Autodesk Inventor part; units mm, degrees
(part 2 of 6)
sketch "Sketch12" plane through (0, 3.175, 0) normal (0, 1, 0) x (1, 0, 0)
  line L0 (-268.616, -146.05) -> (-292.4704, -146.05) projected
  line L1 (-292.4704, -146.05) -> (-280.5432, -134.1228) projected
  line L2 (-280.5432, -134.1228) -> (-268.616, -146.05) projected
  line L3 (-182.1196, -79.5228) -> (-204.0314, -101.4346) projected
  line L4 (-204.0314, -101.4346) -> (-225.9432, -79.5228) projected
  line L5 (-225.9432, -79.5228) -> (-204.0314, -57.611) projected
  line L6 (-204.0314, -57.611) -> (-182.1196, -79.5228) projected
  line L7 (-222.25, -146.05) -> (-241.4626, -146.05) projected
  line L8 (-241.4626, -146.05) -> (-229.5353, -134.1228) projected
  line L9 (-229.5353, -134.1228) -> (-217.4573, -146.2009) projected
  arc A0 (-217.4573, -146.2009) -> (-222.25, -146.05) centre (-222.25, -222.25) ccw projected
  arc A1 (-149.4183, -199.8451) -> (-165.1681, -171.7713) centre (-222.25, -222.25) ccw projected
  line L10 (-165.1681, -171.7713) -> (-153.0236, -159.6267) projected
  line L11 (-153.0236, -159.6267) -> (-131.1117, -181.5385) projected
  line L12 (-131.1117, -181.5385) -> (-149.4183, -199.8451) projected
  line L13 (-25.5039, -185.1306) -> (-3.5921, -207.0425) projected
  line L14 (-3.5921, -207.0425) -> (-25.5039, -228.9543) projected
  line L15 (-25.5039, -228.9543) -> (-47.4158, -207.0425) projected
  line L16 (-47.4158, -207.0425) -> (-25.5039, -185.1306) projected
  line L17 (0, -203.4504) -> (-21.9118, -181.5385) projected
  line L18 (-21.9118, -181.5385) -> (0, -159.6267) projected
  line L19 (0, -159.6267) -> (21.9118, -181.5385) projected
  line L20 (21.9118, -181.5385) -> (0, -203.4504) projected
  line L21 (51.0079, -101.4346) -> (29.096, -79.5228) projected
  line L22 (29.096, -79.5228) -> (51.0079, -57.611) projected
  line L23 (51.0079, -57.611) -> (72.9197, -79.5228) projected
  line L24 (72.9197, -79.5228) -> (51.0079, -101.4346) projected
  line L25 (-102.0157, -159.6267) -> (-80.1039, -181.5385) projected
  line L26 (-80.1039, -181.5385) -> (-102.0157, -203.4504) projected
  line L27 (-102.0157, -203.4504) -> (-123.9275, -181.5385) projected
  line L28 (-123.9275, -181.5385) -> (-102.0157, -159.6267) projected
  line L29 (-102.0157, -210.6346) -> (-80.1039, -232.5464) projected
  line L30 (-80.1039, -232.5464) -> (-102.0157, -254.4582) projected
  line L31 (-102.0157, -254.4582) -> (-123.9275, -232.5464) projected
  line L32 (-123.9275, -232.5464) -> (-102.0157, -210.6346) projected
  line L33 (-25.5039, -236.1385) -> (-3.5921, -258.0503) projected
  line L34 (-3.5921, -258.0503) -> (-25.5039, -279.9621) projected
  line L35 (-25.5039, -279.9621) -> (-47.4158, -258.0503) projected
  line L36 (-47.4158, -258.0503) -> (-25.5039, -236.1385) projected
  line L37 (-146.0075, -298.45) -> (-146.05, -298.45) projected
  line L38 (-146.05, -298.45) -> (-146.05, -268.616) projected
  line L39 (-146.05, -268.616) -> (-131.1117, -283.5542) projected
  line L40 (-131.1117, -283.5542) -> (-146.0075, -298.45) projected
  line L41 (138.8233, -298.45) -> (116.216, -298.45) projected
  line L42 (116.216, -298.45) -> (127.5196, -287.1463) projected
  line L43 (127.5196, -287.1463) -> (138.8233, -298.45) projected
  line L44 (87.8154, -298.45) -> (65.2081, -298.45) projected
  line L45 (65.2081, -298.45) -> (76.5118, -287.1463) projected
  line L46 (76.5118, -287.1463) -> (87.8154, -298.45) projected
  line L47 (51.0079, -254.4582) -> (29.096, -232.5464) projected
  line L48 (29.096, -232.5464) -> (51.0079, -210.6346) projected
  line L49 (51.0079, -210.6346) -> (72.9197, -232.5464) projected
  line L50 (72.9197, -232.5464) -> (51.0079, -254.4582) projected
  line L51 (153.0236, -152.4425) -> (131.1117, -130.5307) projected
  line L52 (131.1117, -130.5307) -> (153.0236, -108.6189) projected
  line L53 (153.0236, -108.6189) -> (174.9354, -130.5307) projected
  line L54 (174.9354, -130.5307) -> (153.0236, -152.4425) projected
  line L55 (255.0393, -50.4268) -> (233.1274, -28.515) projected
  line L56 (233.1274, -28.515) -> (255.0393, -6.6031) projected
  line L57 (255.0393, -6.6031) -> (276.9511, -28.515) projected
  line L58 (276.9511, -28.515) -> (255.0393, -50.4268) projected
  line L59 (284.1353, -130.5307) -> (298.45, -116.216) projected
  line L60 (298.45, -116.216) -> (298.45, -144.8454) projected
  line L61 (298.45, -144.8454) -> (284.1353, -130.5307) projected
  line L62 (255.0393, -57.611) -> (276.9511, -79.5228) projected
  line L63 (276.9511, -79.5228) -> (255.0393, -101.4346) projected
  line L64 (255.0393, -101.4346) -> (233.1274, -79.5228) projected
  line L65 (233.1274, -79.5228) -> (255.0393, -57.611) projected
  line L66 (225.9432, -130.5307) -> (209.3187, -147.1553) projected
  arc A2 (209.3187, -147.1553) -> (200.7384, -149.1495) centre (222.25, -222.25) ccw projected
  line L67 (200.7384, -149.1495) -> (182.1196, -130.5307) projected
  line L68 (182.1196, -130.5307) -> (204.0314, -108.6189) projected
  line L69 (204.0314, -108.6189) -> (225.9432, -130.5307) projected
  line L70 (127.5196, -228.9543) -> (105.6078, -207.0425) projected
  line L71 (105.6078, -207.0425) -> (127.5196, -185.1306) projected
  line L72 (127.5196, -185.1306) -> (147.9092, -205.5202) projected
  arc A3 (147.9092, -205.5202) -> (147.1553, -209.3187) centre (222.25, -222.25) ccw projected
  line L73 (147.1553, -209.3187) -> (127.5196, -228.9543) projected
  line L74 (284.1353, 22.4929) -> (298.45, 36.8076) projected
  line L75 (298.45, 36.8076) -> (298.45, 8.1782) projected
  line L76 (298.45, 8.1782) -> (284.1353, 22.4929) projected
  line L77 (222.25, 146.05) -> (247.4846, 146.05) projected
  line L78 (247.4846, 146.05) -> (229.5353, 128.1007) projected
  line L79 (229.5353, 128.1007) -> (210.7066, 146.9294) projected
  arc A4 (210.7066, 146.9294) -> (222.25, 146.05) centre (222.25, 222.25) ccw projected
  line L80 (255.0393, 51.5889) -> (233.1274, 73.5007) projected
  line L81 (233.1274, 73.5007) -> (255.0393, 95.4126) projected
  line L82 (255.0393, 95.4126) -> (276.9511, 73.5007) projected
  line L83 (276.9511, 73.5007) -> (255.0393, 51.5889) projected
  line L84 (204.0246, 51.5957) -> (182.1196, 73.5007) projected
  line L85 (182.1196, 73.5007) -> (204.0314, 95.4126) projected
  line L86 (204.0314, 95.4126) -> (225.9331, 73.5109) projected
  line L87 (225.9331, 73.5109) -> (204.0246, 51.5957) projected
  line L88 (204.0314, 0.5811) -> (182.1196, 22.4929) projected
  line L89 (182.1196, 22.4929) -> (204.0314, 44.4047) projected
  line L90 (204.0314, 44.4047) -> (225.9432, 22.4929) projected
  line L91 (225.9432, 22.4929) -> (204.0314, 0.5811) projected
  line L92 (178.5275, -32.1071) -> (200.4393, -54.0189) projected
  line L93 (200.4393, -54.0189) -> (178.5275, -75.9307) projected
  line L94 (178.5275, -75.9307) -> (156.6157, -54.0189) projected
  line L95 (156.6157, -54.0189) -> (178.5275, -32.1071) projected
  line L96 (102.0157, -6.6031) -> (123.9275, -28.515) projected
  line L97 (123.9275, -28.515) -> (102.0157, -50.4268) projected
  line L98 (102.0157, -50.4268) -> (80.1039, -28.515) projected
  line L99 (80.1039, -28.515) -> (102.0157, -6.6031) projected
  line L100 (51.0079, -50.4268) -> (29.096, -28.515) projected
  line L101 (29.096, -28.515) -> (51.0079, -6.6031) projected
  line L102 (51.0079, -6.6031) -> (72.9197, -28.515) projected
  line L103 (72.9197, -28.515) -> (51.0079, -50.4268) projected
  line L104 (127.5196, 77.0928) -> (105.6078, 99.0047) projected
  line L105 (105.6078, 99.0047) -> (127.5196, 120.9165) projected
  line L106 (127.5196, 120.9165) -> (149.4315, 99.0047) projected
  line L107 (149.4315, 99.0047) -> (127.5196, 77.0928) projected
  line L108 (153.0236, 102.5968) -> (131.1117, 124.5086) projected
  line L109 (131.1117, 124.5086) -> (153.0236, 146.4204) projected
  line L110 (153.0236, 146.4204) -> (174.9354, 124.5086) projected
  line L111 (174.9354, 124.5086) -> (153.0236, 102.5968) projected
  line L112 (51.0079, 95.4126) -> (72.9197, 73.5007) projected
  line L113 (72.9197, 73.5007) -> (51.0079, 51.5889) projected
  line L114 (51.0079, 51.5889) -> (29.096, 73.5007) projected
  line L115 (29.096, 73.5007) -> (51.0079, 95.4126) projected
  arc A5 (150.9531, 195.3578) -> (168.0787, 168.6598) centre (222.25, 222.25) ccw projected
  line L116 (168.0787, 168.6598) -> (153.0236, 153.6046) projected
  line L117 (153.0236, 153.6046) -> (131.1117, 175.5165) projected
  line L118 (131.1117, 175.5165) -> (150.9531, 195.3578) projected
  line L119 (29.096, 175.5165) -> (51.0079, 197.4283) projected
  line L120 (51.0079, 197.4283) -> (72.9197, 175.5165) projected
  line L121 (72.9197, 175.5165) -> (51.0079, 153.6046) projected
  line L122 (51.0079, 153.6046) -> (29.096, 175.5165) projected
  line L123 (102.0157, 248.4361) -> (123.9275, 226.5243) projected
  line L124 (123.9275, 226.5243) -> (102.0157, 204.6125) projected
  line L125 (102.0157, 204.6125) -> (80.1039, 226.5243) projected
  line L126 (80.1039, 226.5243) -> (102.0157, 248.4361) projected
  line L127 (25.5039, 120.9165) -> (47.4158, 99.0047) projected
  line L128 (47.4158, 99.0047) -> (25.5039, 77.0928) projected
  line L129 (25.5039, 77.0928) -> (3.5921, 99.0047) projected
  line L130 (3.5921, 99.0047) -> (25.5039, 120.9165) projected
  line L131 (76.5118, -177.9464) -> (54.6, -156.0346) projected
  line L132 (54.6, -156.0346) -> (76.5118, -134.1228) projected
  line L133 (76.5118, -134.1228) -> (98.4236, -156.0346) projected
  line L134 (98.4236, -156.0346) -> (76.5118, -177.9464) projected
  line L135 (110.1939, 298.45) -> (144.8454, 298.45) projected
  line L136 (144.8454, 298.45) -> (127.5196, 281.1243) projected
  line L137 (127.5196, 281.1243) -> (110.1939, 298.45) projected
  line L138 (59.186, 298.45) -> (93.8375, 298.45) projected
  line L139 (93.8375, 298.45) -> (76.5118, 281.1243) projected
  line L140 (76.5118, 281.1243) -> (59.186, 298.45) projected
  line L141 (8.1782, 298.45) -> (42.8297, 298.45) projected
  line L142 (42.8297, 298.45) -> (25.5039, 281.1243) projected
  line L143 (25.5039, 281.1243) -> (8.1782, 298.45) projected
  line L144 (-50.0139, 298.45) -> (-29.096, 277.5322) projected
  line L145 (-29.096, 277.5322) -> (-51.0079, 255.6203) projected
  line L146 (-51.0079, 255.6203) -> (-72.9197, 277.5322) projected
  line L147 (-72.9197, 277.5322) -> (-52.0018, 298.45) projected
  line L148 (-52.0018, 298.45) -> (-50.0139, 298.45) projected
  line L149 (-131.1117, 277.5322) -> (-146.05, 262.5939) projected
  line L150 (-146.05, 262.5939) -> (-146.05, 292.4704) projected
  line L151 (-146.05, 292.4704) -> (-131.1117, 277.5322) projected
  line L152 (-51.0079, 204.6125) -> (-72.9197, 226.5243) projected
  line L153 (-72.9197, 226.5243) -> (-51.0079, 248.4361) projected
  line L154 (-51.0079, 248.4361) -> (-29.096, 226.5243) projected
  line L155 (-29.096, 226.5243) -> (-51.0079, 204.6125) projected
  line L156 (-153.0236, 153.6046) -> (-168.0787, 168.6598) projected
  arc A6 (-168.0787, 168.6598) -> (-150.9531, 195.3578) centre (-222.25, 222.25) ccw projected
  line L157 (-150.9531, 195.3578) -> (-131.1117, 175.5165) projected
  line L158 (-131.1117, 175.5165) -> (-153.0236, 153.6046) projected
  line L159 (-76.5118, 171.9243) -> (-54.6, 150.0125) projected
  line L160 (-54.6, 150.0125) -> (-76.5118, 128.1007) projected
  line L161 (-76.5118, 128.1007) -> (-98.4236, 150.0125) projected
  line L162 (-98.4236, 150.0125) -> (-76.5118, 171.9243) projected
  line L163 (-98.4236, 99.0047) -> (-76.5118, 120.9165) projected
  line L164 (-76.5118, 120.9165) -> (-54.6, 99.0047) projected
  line L165 (-54.6, 99.0047) -> (-76.5118, 77.0928) projected
  line L166 (-76.5118, 77.0928) -> (-98.4236, 99.0047) projected
  line L167 (-204.0314, 146.4204) -> (-182.1196, 124.5086) projected
  line L168 (-182.1196, 124.5086) -> (-204.0314, 102.5968) projected
  line L169 (-204.0314, 102.5968) -> (-225.9432, 124.5086) projected
  line L170 (-225.9432, 124.5086) -> (-204.0314, 146.4204) projected
  line L171 (-102.0157, 95.4126) -> (-80.1039, 73.5007) projected
  line L172 (-80.1039, 73.5007) -> (-102.0157, 51.5889) projected
  line L173 (-102.0157, 51.5889) -> (-123.9275, 73.5007) projected
  line L174 (-123.9275, 73.5007) -> (-102.0157, 95.4126) projected
  line L175 (-29.096, 73.5007) -> (-51.0079, 51.5889) projected
  line L176 (-51.0079, 51.5889) -> (-72.9197, 73.5007) projected
  line L177 (-72.9197, 73.5007) -> (-51.0079, 95.4126) projected
  line L178 (-51.0079, 95.4126) -> (-29.096, 73.5007) projected
  line L179 (0, 44.4047) -> (21.9118, 22.4929) projected
  line L180 (21.9118, 22.4929) -> (0, 0.5811) projected
  line L181 (0, 0.5811) -> (-21.9118, 22.4929) projected
  line L182 (-21.9118, 22.4929) -> (0, 44.4047) projected
  line L183 (-25.5039, -83.1149) -> (-3.5921, -105.0267) projected
  line L184 (-3.5921, -105.0267) -> (-25.5039, -126.9386) projected
  line L185 (-25.5039, -126.9386) -> (-47.4158, -105.0267) projected
  line L186 (-47.4158, -105.0267) -> (-25.5039, -83.1149) projected
  line L187 (-76.5118, -24.9229) -> (-98.4236, -3.011) projected
  line L188 (-98.4236, -3.011) -> (-76.5118, 18.9008) projected
  line L189 (-76.5118, 18.9008) -> (-54.6, -3.011) projected
  line L190 (-54.6, -3.011) -> (-76.5118, -24.9229) projected
  line L191 (-153.0236, 44.4047) -> (-131.1117, 22.4929) projected
  line L192 (-131.1117, 22.4929) -> (-153.0236, 0.5811) projected
  line L193 (-153.0236, 0.5811) -> (-159.5933, 7.1508) projected
  line L194 (-159.5933, 7.1508) -> (-174.933, 22.4952) projected
  line L195 (-174.933, 22.4952) -> (-153.0236, 44.4047) projected
  line L196 (-76.5118, -126.9386) -> (-98.4236, -105.0267) projected
  line L197 (-98.4236, -105.0267) -> (-76.5118, -83.1149) projected
  line L198 (-76.5118, -83.1149) -> (-54.6, -105.0267) projected
  line L199 (-54.6, -105.0267) -> (-76.5118, -126.9386) projected
  line L200 (3.5921, 201.0204) -> (25.5039, 222.9322) projected
  line L201 (25.5039, 222.9322) -> (47.4158, 201.0204) projected
  line L202 (47.4158, 201.0204) -> (25.5039, 179.1086) projected
  line L203 (25.5039, 179.1086) -> (3.5921, 201.0204) projected
  line L204 (-298.45, 146.05) -> (-262.5939, 146.05) projected
  line L205 (-262.5939, 146.05) -> (-280.5247, 128.1192) projected
  line L206 (-280.5247, 128.1192) -> (-298.45, 146.05) projected
  line L207 (-229.5353, 120.9165) -> (-207.6235, 99.0047) projected
  line L208 (-207.6235, 99.0047) -> (-229.5246, 77.1035) projected
  line L209 (-229.5246, 77.1035) -> (-251.4331, 99.0187) projected
  line L210 (-251.4331, 99.0187) -> (-229.5353, 120.9165) projected
  line L211 (-229.5353, 69.9086) -> (-207.6235, 47.9968) projected
  line L212 (-207.6235, 47.9968) -> (-229.5353, 26.085) projected
  line L213 (-229.5353, 26.085) -> (-251.4472, 47.9968) projected
  line L214 (-251.4472, 47.9968) -> (-229.5353, 69.9086) projected
  line L215 (-284.1353, 22.4929) -> (-298.45, 8.1782) projected
  line L216 (-298.45, 8.1782) -> (-298.45, 36.8076) projected
  line L217 (-298.45, 36.8076) -> (-284.1353, 22.4929) projected
  line L218 (-225.9432, -28.515) -> (-204.0314, -6.6031) projected
  line L219 (-204.0314, -6.6031) -> (-182.1196, -28.515) projected
  line L220 (-182.1196, -28.515) -> (-204.0314, -50.4268) projected
  line L221 (-204.0314, -50.4268) -> (-225.9432, -28.515) projected
  line L222 (-280.5432, -32.1071) -> (-258.6314, -54.0189) projected
  line L223 (-258.6314, -54.0189) -> (-280.5432, -75.9307) projected
  line L224 (-280.5432, -75.9307) -> (-298.45, -58.0239) projected
  line L225 (-298.45, -58.0239) -> (-298.45, -50.0139) projected
  line L226 (-298.45, -50.0139) -> (-280.5432, -32.1071) projected
  line L227 (-251.4472, -54.0189) -> (-229.5353, -32.1071) projected
  line L228 (-229.5353, -32.1071) -> (-207.6235, -54.0189) projected
  line L229 (-207.6235, -54.0189) -> (-229.5353, -75.9307) projected
  line L230 (-229.5353, -75.9307) -> (-251.4472, -54.0189) projected
  line L231 (-229.5353, 18.9008) -> (-207.6235, -3.011) projected
  line L232 (-207.6235, -3.011) -> (-229.5353, -24.9229) projected
  line L233 (-229.5353, -24.9229) -> (-251.4472, -3.011) projected
  line L234 (-251.4472, -3.011) -> (-229.5353, 18.9008) projected
  line L235 (-284.1353, 73.5007) -> (-298.45, 59.186) projected
  line L236 (-298.45, 59.186) -> (-298.45, 87.8154) projected
  line L237 (-298.45, 87.8154) -> (-284.1353, 73.5007) projected
  line L238 (-204.0314, 44.4047) -> (-182.1196, 22.4929) projected
  line L239 (-182.1196, 22.4929) -> (-204.0314, 0.5811) projected
  line L240 (-204.0314, 0.5811) -> (-225.9432, 22.4929) projected
  line L241 (-225.9432, 22.4929) -> (-204.0314, 44.4047) projected
  line L242 (-255.0393, 95.4126) -> (-233.1274, 73.5007) projected
  line L243 (-233.1274, 73.5007) -> (-255.0393, 51.5889) projected
  line L244 (-255.0393, 51.5889) -> (-276.9511, 73.5007) projected
  line L245 (-276.9511, 73.5007) -> (-255.0393, 95.4126) projected
  line L246 (-254.6689, 146.05) -> (-233.1274, 124.5086) projected
  line L247 (-233.1274, 124.5086) -> (-255.0247, 102.6114) projected
  line L248 (-255.0247, 102.6114) -> (-276.9331, 124.5266) projected
  line L249 (-276.9331, 124.5266) -> (-255.4097, 146.05) projected
  line L250 (-255.4097, 146.05) -> (-254.6689, 146.05) projected
  line L251 (-25.5039, 179.1086) -> (-47.4158, 201.0204) projected
  line L252 (-47.4158, 201.0204) -> (-25.5039, 222.9322) projected
  line L253 (-25.5039, 222.9322) -> (-3.5921, 201.0204) projected
  line L254 (-3.5921, 201.0204) -> (-25.5039, 179.1086) projected
  line L255 (-102.0157, -101.4346) -> (-123.9275, -79.5228) projected
  line L256 (-123.9275, -79.5228) -> (-102.0157, -57.611) projected
  line L257 (-102.0157, -57.611) -> (-80.1039, -79.5228) projected
  line L258 (-80.1039, -79.5228) -> (-102.0157, -101.4346) projected
  line L259 (-105.6078, -3.011) -> (-127.5196, -24.9229) projected
  line L260 (-127.5196, -24.9229) -> (-149.4315, -3.011) projected
  line L261 (-149.4315, -3.011) -> (-127.5196, 18.9008) projected
  line L262 (-127.5196, 18.9008) -> (-105.6078, -3.011) projected
  line L263 (-51.0079, 0.5811) -> (-72.9197, 22.4929) projected
  line L264 (-72.9197, 22.4929) -> (-51.0079, 44.4047) projected
  line L265 (-51.0079, 44.4047) -> (-29.096, 22.4929) projected
  line L266 (-29.096, 22.4929) -> (-51.0079, 0.5811) projected
  line L267 (-25.5039, -75.9307) -> (-47.4158, -54.0189) projected
  line L268 (-47.4158, -54.0189) -> (-25.5039, -32.1071) projected
  line L269 (-25.5039, -32.1071) -> (-3.5921, -54.0189) projected
  line L270 (-3.5921, -54.0189) -> (-25.5039, -75.9307) projected
  line L271 (25.5039, 69.9086) -> (47.4158, 47.9968) projected
  line L272 (47.4158, 47.9968) -> (25.5039, 26.085) projected
  line L273 (25.5039, 26.085) -> (3.5921, 47.9968) projected
  line L274 (3.5921, 47.9968) -> (25.5039, 69.9086) projected
  line L275 (-3.5921, 99.0047) -> (-25.5039, 77.0928) projected
  line L276 (-25.5039, 77.0928) -> (-47.4158, 99.0047) projected
  line L277 (-47.4158, 99.0047) -> (-25.5039, 120.9165) projected
  line L278 (-25.5039, 120.9165) -> (-3.5921, 99.0047) projected
  line L279 (-149.4315, 47.9968) -> (-127.5196, 69.9086) projected
  line L280 (-127.5196, 69.9086) -> (-105.6078, 47.9968) projected
  line L281 (-105.6078, 47.9968) -> (-127.5196, 26.085) projected
  line L282 (-127.5196, 26.085) -> (-149.4315, 47.9968) projected
  line L283 (-171.7713, 165.1681) -> (-156.6157, 150.0125) projected
  line L284 (-156.6157, 150.0125) -> (-178.5275, 128.1007) projected
  line L285 (-178.5275, 128.1007) -> (-199.8451, 149.4183) projected
  arc A7 (-199.8451, 149.4183) -> (-171.7713, 165.1681) centre (-222.25, 222.25) ccw projected
  line L286 (-72.9197, 124.5086) -> (-51.0079, 146.4204) projected
  line L287 (-51.0079, 146.4204) -> (-29.096, 124.5086) projected
  line L288 (-29.096, 124.5086) -> (-51.0079, 102.5968) projected
  line L289 (-51.0079, 102.5968) -> (-72.9197, 124.5086) projected
  line L290 (-102.0157, 102.5968) -> (-123.9275, 124.5086) projected
  line L291 (-123.9275, 124.5086) -> (-102.0157, 146.4204) projected
  line L292 (-102.0157, 146.4204) -> (-80.1039, 124.5086) projected
  line L293 (-80.1039, 124.5086) -> (-102.0157, 102.5968) projected
  arc A8 (-146.9294, 210.7066) -> (-146.05, 222.25) centre (-222.25, 222.25) ccw projected
  line L294 (-146.05, 222.25) -> (-146.05, 241.4626) projected
  line L295 (-146.05, 241.4626) -> (-131.1117, 226.5243) projected
  line L296 (-131.1117, 226.5243) -> (-146.9294, 210.7066) projected
  line L297 (-76.5118, 230.1164) -> (-98.4236, 252.0282) projected
  line L298 (-98.4236, 252.0282) -> (-76.5118, 273.9401) projected
  line L299 (-76.5118, 273.9401) -> (-54.6, 252.0282) projected
  line L300 (-54.6, 252.0282) -> (-76.5118, 230.1164) projected
  line L301 (-144.8454, 298.45) -> (-110.1939, 298.45) projected
  line L302 (-110.1939, 298.45) -> (-127.5196, 281.1243) projected
  line L303 (-127.5196, 281.1243) -> (-144.8454, 298.45) projected
  line L304 (-42.8297, 298.45) -> (-8.1782, 298.45) projected
  line L305 (-8.1782, 298.45) -> (-25.5039, 281.1243) projected
  line L306 (-25.5039, 281.1243) -> (-42.8297, 298.45) projected
  line L307 (-21.9118, 277.5322) -> (-0.994, 298.45) projected
  line L308 (-0.994, 298.45) -> (0.994, 298.45) projected
  line L309 (0.994, 298.45) -> (21.9118, 277.5322) projected
  line L310 (21.9118, 277.5322) -> (0, 255.6203) projected
  line L311 (0, 255.6203) -> (-21.9118, 277.5322) projected
  line L312 (52.0018, 298.45) -> (72.9197, 277.5322) projected
  line L313 (72.9197, 277.5322) -> (51.0079, 255.6203) projected
  line L314 (51.0079, 255.6203) -> (29.096, 277.5322) projected
  line L315 (29.096, 277.5322) -> (50.0139, 298.45) projected
  line L316 (50.0139, 298.45) -> (52.0018, 298.45) projected
  line L317 (131.1117, 277.5322) -> (146.05, 292.4704) projected
  line L318 (146.05, 292.4704) -> (146.05, 262.5939) projected
  line L319 (146.05, 262.5939) -> (131.1117, 277.5322) projected
  line L320 (76.5118, -126.9386) -> (54.6, -105.0267) projected
  line L321 (54.6, -105.0267) -> (76.5118, -83.1149) projected
  line L322 (76.5118, -83.1149) -> (98.4236, -105.0267) projected
  line L323 (98.4236, -105.0267) -> (76.5118, -126.9386) projected
  line L324 (105.6078, 252.0282) -> (127.5196, 273.9401) projected
  line L325 (127.5196, 273.9401) -> (146.05, 255.4097) projected
  line L326 (146.05, 255.4097) -> (146.05, 248.6468) projected
  line L327 (146.05, 248.6468) -> (127.5196, 230.1164) projected
  line L328 (127.5196, 230.1164) -> (105.6078, 252.0282) projected
  line L329 (54.6, 201.0204) -> (76.5118, 222.9322) projected
  line L330 (76.5118, 222.9322) -> (98.4236, 201.0204) projected
  line L331 (98.4236, 201.0204) -> (76.5118, 179.1086) projected
  line L332 (76.5118, 179.1086) -> (54.6, 201.0204) projected
  line L333 (76.5118, 128.1007) -> (54.6, 150.0125) projected
  line L334 (54.6, 150.0125) -> (76.5118, 171.9243) projected
  line L335 (76.5118, 171.9243) -> (98.4236, 150.0125) projected
  line L336 (98.4236, 150.0125) -> (76.5118, 128.1007) projected
  arc A9 (171.7713, 165.1681) -> (199.8451, 149.4183) centre (222.25, 222.25) ccw projected
  line L337 (199.8451, 149.4183) -> (178.5275, 128.1007) projected
  line L338 (178.5275, 128.1007) -> (156.6157, 150.0125) projected
  line L339 (156.6157, 150.0125) -> (171.7713, 165.1681) projected
  line L340 (51.0079, 146.4204) -> (72.9197, 124.5086) projected
  line L341 (72.9197, 124.5086) -> (51.0079, 102.5968) projected
  line L342 (51.0079, 102.5968) -> (29.096, 124.5086) projected
  line L343 (29.096, 124.5086) -> (51.0079, 146.4204) projected
  line L344 (204.0314, 102.5968) -> (182.1196, 124.5086) projected
  line L345 (182.1196, 124.5086) -> (204.0314, 146.4204) projected
  line L346 (204.0314, 146.4204) -> (225.9432, 124.5086) projected
  line L347 (225.9432, 124.5086) -> (204.0314, 102.5968) projected
  line L348 (102.0157, 95.4126) -> (123.9275, 73.5007) projected
  line L349 (123.9275, 73.5007) -> (102.0157, 51.5889) projected
  line L350 (102.0157, 51.5889) -> (80.1039, 73.5007) projected
  line L351 (80.1039, 73.5007) -> (102.0157, 95.4126) projected
  line L352 (76.5118, 18.9008) -> (98.4236, -3.011) projected
  line L353 (98.4236, -3.011) -> (76.5118, -24.9229) projected
  line L354 (76.5118, -24.9229) -> (54.6, -3.011) projected
  line L355 (54.6, -3.011) -> (76.5118, 18.9008) projected
  line L356 (127.5196, 18.9008) -> (149.4315, -3.011) projected
  line L357 (149.4315, -3.011) -> (127.5196, -24.9229) projected
  line L358 (127.5196, -24.9229) -> (105.6078, -3.011) projected
  line L359 (105.6078, -3.011) -> (127.5196, 18.9008) projected
  line L360 (127.5196, -32.1071) -> (149.4315, -54.0189) projected
  line L361 (149.4315, -54.0189) -> (127.5196, -75.9307) projected
  line L362 (127.5196, -75.9307) -> (105.6078, -54.0189) projected
  line L363 (105.6078, -54.0189) -> (127.5196, -32.1071) projected
  line L364 (204.0314, -6.6031) -> (225.9432, -28.515) projected
  line L365 (225.9432, -28.515) -> (204.0314, -50.4268) projected
  line L366 (204.0314, -50.4268) -> (182.1196, -28.515) projected
  line L367 (182.1196, -28.515) -> (204.0314, -6.6031) projected
  line L368 (229.5353, 26.085) -> (207.6235, 47.9968) projected
  line L369 (207.6235, 47.9968) -> (229.5353, 69.9086) projected
  line L370 (229.5353, 69.9086) -> (251.4472, 47.9968) projected
  line L371 (251.4472, 47.9968) -> (229.5353, 26.085) projected
  line L372 (229.5246, 77.1035) -> (207.6235, 99.0047) projected
  line L373 (207.6235, 99.0047) -> (229.5353, 120.9165) projected
  line L374 (229.5353, 120.9165) -> (251.4331, 99.0187) projected
  line L375 (251.4331, 99.0187) -> (229.5246, 77.1035) projected
  line L376 (262.5939, 146.05) -> (298.45, 146.05) projected
  line L377 (298.45, 146.05) -> (280.5247, 128.1192) projected
  line L378 (280.5247, 128.1192) -> (262.5939, 146.05) projected
  line L379 (-14.2003, -298.45) -> (-36.8076, -298.45) projected
  line L380 (-36.8076, -298.45) -> (-25.5039, -287.1463) projected
  line L381 (-25.5039, -287.1463) -> (-14.2003, -298.45) projected
  arc A10 (146.2009, -217.4573) -> (146.05, -222.25) centre (222.25, -222.25) ccw projected
  line L382 (146.05, -222.25) -> (146.05, -247.4846) projected
  line L383 (146.05, -247.4846) -> (131.1117, -232.5464) projected
  line L384 (131.1117, -232.5464) -> (146.2009, -217.4573) projected
  line L385 (229.5353, -83.1149) -> (251.4472, -105.0267) projected
  line L386 (251.4472, -105.0267) -> (229.5353, -126.9386) projected
  line L387 (229.5353, -126.9386) -> (207.6235, -105.0267) projected
  line L388 (207.6235, -105.0267) -> (229.5353, -83.1149) projected
  line L389 (276.9511, -130.5307) -> (261.4318, -146.05) projected
  line L390 (261.4318, -146.05) -> (248.6468, -146.05) projected
  line L391 (248.6468, -146.05) -> (233.1274, -130.5307) projected
  line L392 (233.1274, -130.5307) -> (255.0393, -108.6189) projected
  line L393 (255.0393, -108.6189) -> (276.9511, -130.5307) projected
  line L394 (284.1353, -79.5228) -> (298.45, -65.2081) projected
  line L395 (298.45, -65.2081) -> (298.45, -93.8375) projected
  line L396 (298.45, -93.8375) -> (284.1353, -79.5228) projected
  line L397 (229.5353, -32.1071) -> (251.4472, -54.0189) projected
  line L398 (251.4472, -54.0189) -> (229.5353, -75.9307) projected
  line L399 (229.5353, -75.9307) -> (207.6235, -54.0189) projected
  line L400 (207.6235, -54.0189) -> (229.5353, -32.1071) projected
  line L401 (127.5196, -177.9464) -> (105.6078, -156.0346) projected
  line L402 (105.6078, -156.0346) -> (127.5196, -134.1228) projected
  line L403 (127.5196, -134.1228) -> (149.4315, -156.0346) projected
  line L404 (149.4315, -156.0346) -> (127.5196, -177.9464) projected
  line L405 (25.5039, -236.1385) -> (47.4158, -258.0503) projected
  line L406 (47.4158, -258.0503) -> (25.5039, -279.9621) projected
  line L407 (25.5039, -279.9621) -> (3.5921, -258.0503) projected
  line L408 (3.5921, -258.0503) -> (25.5039, -236.1385) projected
  line L409 (76.5118, -279.9621) -> (54.6, -258.0503) projected
  line L410 (54.6, -258.0503) -> (76.5118, -236.1385) projected
  line L411 (76.5118, -236.1385) -> (98.4236, -258.0503) projected
  line L412 (98.4236, -258.0503) -> (76.5118, -279.9621) projected
  line L413 (146.05, -268.616) -> (146.05, -298.45) projected
  line L414 (146.05, -298.45) -> (146.0075, -298.45) projected
  line L415 (146.0075, -298.45) -> (131.1117, -283.5542) projected
  line L416 (131.1117, -283.5542) -> (146.05, -268.616) projected
  line L417 (-109.0318, -298.45) -> (-123.9275, -283.5542) projected
  line L418 (-123.9275, -283.5542) -> (-102.0157, -261.6424) projected
  line L419 (-102.0157, -261.6424) -> (-80.1039, -283.5542) projected
  line L420 (-80.1039, -283.5542) -> (-94.9996, -298.45) projected
  line L421 (-94.9996, -298.45) -> (-109.0318, -298.45) projected
  line L422 (-76.5118, -236.1385) -> (-54.6, -258.0503) projected
  line L423 (-54.6, -258.0503) -> (-76.5118, -279.9621) projected
  line L424 (-76.5118, -279.9621) -> (-98.4236, -258.0503) projected
  line L425 (-98.4236, -258.0503) -> (-76.5118, -236.1385) projected
  line L426 (-146.05, -261.4318) -> (-146.05, -254.6689) projected
  line L427 (-146.05, -254.6689) -> (-127.5196, -236.1385) projected
  line L428 (-127.5196, -236.1385) -> (-105.6078, -258.0503) projected
  line L429 (-105.6078, -258.0503) -> (-127.5196, -279.9621) projected
  line L430 (-127.5196, -279.9621) -> (-146.05, -261.4318) projected
  line L431 (-25.5039, -177.9464) -> (-47.4158, -156.0346) projected
  line L432 (-47.4158, -156.0346) -> (-25.5039, -134.1228) projected
  line L433 (-25.5039, -134.1228) -> (-3.5921, -156.0346) projected
  line L434 (-3.5921, -156.0346) -> (-25.5039, -177.9464) projected
  line L435 (25.5039, -75.9307) -> (3.5921, -54.0189) projected
  line L436 (3.5921, -54.0189) -> (25.5039, -32.1071) projected
  line L437 (25.5039, -32.1071) -> (47.4158, -54.0189) projected
  line L438 (47.4158, -54.0189) -> (25.5039, -75.9307) projected
  line L439 (25.5039, -228.9543) -> (3.5921, -207.0425) projected
  line L440 (3.5921, -207.0425) -> (25.5039, -185.1306) projected
  line L441 (25.5039, -185.1306) -> (47.4158, -207.0425) projected
  line L442 (47.4158, -207.0425) -> (25.5039, -228.9543) projected
  line L443 (-51.0079, -159.6267) -> (-29.096, -181.5385) projected
  line L444 (-29.096, -181.5385) -> (-51.0079, -203.4504) projected
  line L445 (-51.0079, -203.4504) -> (-72.9197, -181.5385) projected
  line L446 (-72.9197, -181.5385) -> (-51.0079, -159.6267) projected
  line L447 (-127.5196, -134.1228) -> (-105.6078, -156.0346) projected
  line L448 (-105.6078, -156.0346) -> (-127.5196, -177.9464) projected
  line L449 (-127.5196, -177.9464) -> (-149.4315, -156.0346) projected
  line L450 (-149.4315, -156.0346) -> (-127.5196, -134.1228) projected
  line L451 (-182.1196, -130.5307) -> (-200.7384, -149.1495) projected
  arc A11 (-200.7384, -149.1495) -> (-209.3187, -147.1553) centre (-222.25, -222.25) ccw projected
  line L452 (-209.3187, -147.1553) -> (-225.9432, -130.5307) projected
  line L453 (-225.9432, -130.5307) -> (-204.0314, -108.6189) projected
  line L454 (-204.0314, -108.6189) -> (-182.1196, -130.5307) projected
  line L455 (-207.6235, -105.0267) -> (-229.5353, -126.9386) projected
  line L456 (-229.5353, -126.9386) -> (-251.4472, -105.0267) projected
  line L457 (-251.4472, -105.0267) -> (-229.5353, -83.1149) projected
  line L458 (-229.5353, -83.1149) -> (-207.6235, -105.0267) projected
  line L459 (-233.1274, -130.5307) -> (-248.6468, -146.05) projected
  line L460 (-248.6468, -146.05) -> (-261.4318, -146.05) projected
  line L461 (-261.4318, -146.05) -> (-276.9511, -130.5307) projected
  line L462 (-276.9511, -130.5307) -> (-255.0393, -108.6189) projected
  line L463 (-255.0393, -108.6189) -> (-233.1274, -130.5307) projected
  line L464 (-284.1353, -130.5307) -> (-298.45, -144.8454) projected
  line L465 (-298.45, -144.8454) -> (-298.45, -116.216) projected
  line L466 (-298.45, -116.216) -> (-284.1353, -130.5307) projected
  line L467 (-156.6157, -54.0189) -> (-178.5275, -75.9307) projected
  line L468 (-178.5275, -75.9307) -> (-200.4393, -54.0189) projected
  line L469 (-200.4393, -54.0189) -> (-178.5275, -32.1071) projected
  line L470 (-178.5275, -32.1071) -> (-156.6157, -54.0189) projected
  arc A12 (-168.6598, -168.0787) -> (-195.3578, -150.9531) centre (-222.25, -222.25) ccw projected
  line L471 (-195.3578, -150.9531) -> (-178.5275, -134.1228) projected
  line L472 (-178.5275, -134.1228) -> (-156.6157, -156.0346) projected
  line L473 (-156.6157, -156.0346) -> (-168.6598, -168.0787) projected
  line L474 (-102.0157, -108.6189) -> (-80.1039, -130.5307) projected
  line L475 (-80.1039, -130.5307) -> (-102.0157, -152.4425) projected
  line L476 (-102.0157, -152.4425) -> (-123.9275, -130.5307) projected
  line L477 (-123.9275, -130.5307) -> (-102.0157, -108.6189) projected
  line L478 (0, -254.4582) -> (-21.9118, -232.5464) projected
  line L479 (-21.9118, -232.5464) -> (0, -210.6346) projected
  line L480 (0, -210.6346) -> (21.9118, -232.5464) projected
  line L481 (21.9118, -232.5464) -> (0, -254.4582) projected
  line L482 (0, -152.4425) -> (-21.9118, -130.5307) projected
  line L483 (-21.9118, -130.5307) -> (0, -108.6189) projected
  line L484 (0, -108.6189) -> (21.9118, -130.5307) projected
  line L485 (21.9118, -130.5307) -> (0, -152.4425) projected
  line L486 (25.5039, -126.9386) -> (3.5921, -105.0267) projected
  line L487 (3.5921, -105.0267) -> (25.5039, -83.1149) projected
  line L488 (25.5039, -83.1149) -> (47.4158, -105.0267) projected
  line L489 (47.4158, -105.0267) -> (25.5039, -126.9386) projected
  line L490 (-127.5196, -185.1306) -> (-105.6078, -207.0425) projected
  line L491 (-105.6078, -207.0425) -> (-127.5196, -228.9543) projected
  line L492 (-127.5196, -228.9543) -> (-147.1553, -209.3187) projected
  arc A13 (-147.1553, -209.3187) -> (-147.9092, -205.5202) centre (-222.25, -222.25) ccw projected
  line L493 (-147.9092, -205.5202) -> (-127.5196, -185.1306) projected
  line L494 (-76.5118, -185.1306) -> (-54.6, -207.0425) projected
  line L495 (-54.6, -207.0425) -> (-76.5118, -228.9543) projected
  line L496 (-76.5118, -228.9543) -> (-98.4236, -207.0425) projected
  line L497 (-98.4236, -207.0425) -> (-76.5118, -185.1306) projected
  line L498 (0, -6.6031) -> (21.9118, -28.515) projected
  line L499 (21.9118, -28.515) -> (0, -50.4268) projected
  line L500 (0, -50.4268) -> (-21.9118, -28.515) projected
  line L501 (-21.9118, -28.515) -> (0, -6.6031) projected
  line L502 (-116.216, -298.45) -> (-138.8233, -298.45) projected
  line L503 (-138.8233, -298.45) -> (-127.5196, -287.1463) projected
  line L504 (-127.5196, -287.1463) -> (-116.216, -298.45) projected
  line L505 (146.05, -254.6689) -> (146.05, -261.4318) projected
  line L506 (146.05, -261.4318) -> (127.5196, -279.9621) projected
  line L507 (127.5196, -279.9621) -> (105.6078, -258.0503) projected
  line L508 (105.6078, -258.0503) -> (127.5196, -236.1385) projected
  line L509 (127.5196, -236.1385) -> (146.05, -254.6689) projected
  line L510 (72.9197, -283.5542) -> (58.0239, -298.45) projected
  line L511 (58.0239, -298.45) -> (43.9918, -298.45) projected
  line L512 (43.9918, -298.45) -> (29.096, -283.5542) projected
  line L513 (29.096, -283.5542) -> (51.0079, -261.6424) projected
  line L514 (51.0079, -261.6424) -> (72.9197, -283.5542) projected
  line L515 (76.5118, -185.1306) -> (98.4236, -207.0425) projected
  line L516 (98.4236, -207.0425) -> (76.5118, -228.9543) projected
  line L517 (76.5118, -228.9543) -> (54.6, -207.0425) projected
  line L518 (54.6, -207.0425) -> (76.5118, -185.1306) projected
  line L519 (178.5275, -83.1149) -> (200.4393, -105.0267) projected
  line L520 (200.4393, -105.0267) -> (178.5275, -126.9386) projected
  line L521 (178.5275, -126.9386) -> (156.6157, -105.0267) projected
  line L522 (156.6157, -105.0267) -> (178.5275, -83.1149) projected
  line L523 (280.5432, -24.9229) -> (258.6314, -3.011) projected
  line L524 (258.6314, -3.011) -> (280.5432, 18.9008) projected
  line L525 (280.5432, 18.9008) -> (298.45, 0.994) projected
  line L526 (298.45, 0.994) -> (298.45, -7.0161) projected
  line L527 (298.45, -7.0161) -> (280.5432, -24.9229) projected
  line L528 (298.45, -101.0217) -> (298.45, -109.0318) projected
  line L529 (298.45, -109.0318) -> (280.5432, -126.9386) projected
  line L530 (280.5432, -126.9386) -> (258.6314, -105.0267) projected
  line L531 (258.6314, -105.0267) -> (280.5432, -83.1149) projected
  line L532 (280.5432, -83.1149) -> (298.45, -101.0217) projected
  line L533 (292.4704, -146.05) -> (268.616, -146.05) projected
  line L534 (268.616, -146.05) -> (280.5432, -134.1228) projected
  line L535 (280.5432, -134.1228) -> (292.4704, -146.05) projected
  line L536 (168.6598, -168.0787) -> (156.6157, -156.0346) projected
  line L537 (156.6157, -156.0346) -> (178.5275, -134.1228) projected
  line L538 (178.5275, -134.1228) -> (195.3578, -150.9531) projected
  arc A14 (195.3578, -150.9531) -> (168.6598, -168.0787) centre (222.25, -222.25) ccw projected
  line L539 (102.0157, -210.6346) -> (123.9275, -232.5464) projected
  line L540 (123.9275, -232.5464) -> (102.0157, -254.4582) projected
  line L541 (102.0157, -254.4582) -> (80.1039, -232.5464) projected
  line L542 (80.1039, -232.5464) -> (102.0157, -210.6346) projected
  line L543 (284.1353, 73.5007) -> (298.45, 87.8154) projected
  line L544 (298.45, 87.8154) -> (298.45, 59.186) projected
  line L545 (298.45, 59.186) -> (284.1353, 73.5007) projected
  line L546 (233.1274, 124.5086) -> (254.6689, 146.05) projected
  line L547 (254.6689, 146.05) -> (255.4097, 146.05) projected
  line L548 (255.4097, 146.05) -> (276.9331, 124.5266) projected
  line L549 (276.9331, 124.5266) -> (255.0247, 102.6114) projected
  line L550 (255.0247, 102.6114) -> (233.1274, 124.5086) projected
  line L551 (280.5432, 26.085) -> (258.6314, 47.9968) projected
  line L552 (258.6314, 47.9968) -> (280.5432, 69.9086) projected
  line L553 (280.5432, 69.9086) -> (298.45, 52.0018) projected
  line L554 (298.45, 52.0018) -> (298.45, 43.9918) projected
  line L555 (298.45, 43.9918) -> (280.5432, 26.085) projected
  line L556 (178.5246, 26.0879) -> (156.6157, 47.9968) projected
  line L557 (156.6157, 47.9968) -> (178.5275, 69.9086) projected
  line L558 (178.5275, 69.9086) -> (200.4331, 48.0031) projected
  line L559 (200.4331, 48.0031) -> (178.5246, 26.0879) projected
  line L560 (178.5275, 18.9008) -> (200.4393, -3.011) projected
  line L561 (200.4393, -3.011) -> (178.5275, -24.9229) projected
  line L562 (178.5275, -24.9229) -> (156.6157, -3.011) projected
  line L563 (156.6157, -3.011) -> (178.5275, 18.9008) projected
  line L564 (153.0236, -57.611) -> (174.9354, -79.5228) projected
  line L565 (174.9354, -79.5228) -> (153.0236, -101.4346) projected
  line L566 (153.0236, -101.4346) -> (131.1117, -79.5228) projected
  line L567 (131.1117, -79.5228) -> (153.0236, -57.611) projected
  line L568 (76.5118, -75.9307) -> (54.6, -54.0189) projected
  line L569 (54.6, -54.0189) -> (76.5118, -32.1071) projected
  line L570 (76.5118, -32.1071) -> (98.4236, -54.0189) projected
  line L571 (98.4236, -54.0189) -> (76.5118, -75.9307) projected
  line L572 (102.0157, 44.4047) -> (123.9275, 22.4929) projected
  line L573 (123.9275, 22.4929) -> (102.0157, 0.5811) projected
  line L574 (102.0157, 0.5811) -> (80.1039, 22.4929) projected
  line L575 (80.1039, 22.4929) -> (102.0157, 44.4047) projected
  line L576 (153.0236, 51.5889) -> (131.1117, 73.5007) projected
  line L577 (131.1117, 73.5007) -> (153.0236, 95.4126) projected
  line L578 (153.0236, 95.4126) -> (174.9354, 73.5007) projected
  line L579 (174.9354, 73.5007) -> (153.0236, 51.5889) projected
  line L580 (102.0157, 102.5968) -> (80.1039, 124.5086) projected
  line L581 (80.1039, 124.5086) -> (102.0157, 146.4204) projected
  line L582 (102.0157, 146.4204) -> (123.9275, 124.5086) projected
  line L583 (123.9275, 124.5086) -> (102.0157, 102.5968) projected
  line L584 (76.5118, 69.9086) -> (98.4236, 47.9968) projected
  line L585 (98.4236, 47.9968) -> (76.5118, 26.085) projected
  line L586 (76.5118, 26.085) -> (54.6, 47.9968) projected
  line L587 (54.6, 47.9968) -> (76.5118, 69.9086) projected
  line L588 (127.5196, 128.1007) -> (105.6078, 150.0125) projected
  line L589 (105.6078, 150.0125) -> (127.5196, 171.9243) projected
  line L590 (127.5196, 171.9243) -> (149.4315, 150.0125) projected
  line L591 (149.4315, 150.0125) -> (127.5196, 128.1007) projected
  line L592 (25.5039, 128.1007) -> (3.5921, 150.0125) projected
  line L593 (3.5921, 150.0125) -> (25.5039, 171.9243) projected
  line L594 (25.5039, 171.9243) -> (47.4158, 150.0125) projected
  line L595 (47.4158, 150.0125) -> (25.5039, 128.1007) projected
  arc A15 (148.9209, 201.531) -> (149.1495, 200.7384) centre (222.25, 222.25) ccw projected
  line L596 (149.1495, 200.7384) -> (127.5196, 179.1086) projected
  line L597 (127.5196, 179.1086) -> (105.6078, 201.0204) projected
  line L598 (105.6078, 201.0204) -> (127.5196, 222.9322) projected
  line L599 (127.5196, 222.9322) -> (148.9209, 201.531) projected
  line L600 (127.5196, -126.9386) -> (105.6078, -105.0267) projected
  line L601 (105.6078, -105.0267) -> (127.5196, -83.1149) projected
  line L602 (127.5196, -83.1149) -> (149.4315, -105.0267) projected
  line L603 (149.4315, -105.0267) -> (127.5196, -126.9386) projected
  line L604 (51.0079, -152.4425) -> (29.096, -130.5307) projected
  line L605 (29.096, -130.5307) -> (51.0079, -108.6189) projected
  line L606 (51.0079, -108.6189) -> (72.9197, -130.5307) projected
  line L607 (72.9197, -130.5307) -> (51.0079, -152.4425) projected
  line L608 (101.0217, 298.45) -> (103.0097, 298.45) projected
  line L609 (103.0097, 298.45) -> (123.9275, 277.5322) projected
  line L610 (123.9275, 277.5322) -> (102.0157, 255.6203) projected
  line L611 (102.0157, 255.6203) -> (80.1039, 277.5322) projected
  line L612 (80.1039, 277.5322) -> (101.0217, 298.45) projected
  line L613 (51.0079, 204.6125) -> (29.096, 226.5243) projected
  line L614 (29.096, 226.5243) -> (51.0079, 248.4361) projected
  line L615 (51.0079, 248.4361) -> (72.9197, 226.5243) projected
  line L616 (72.9197, 226.5243) -> (51.0079, 204.6125) projected
  line L617 (0, 248.4361) -> (21.9118, 226.5243) projected
  line L618 (21.9118, 226.5243) -> (0, 204.6125) projected
  line L619 (0, 204.6125) -> (-21.9118, 226.5243) projected
  line L620 (-21.9118, 226.5243) -> (0, 248.4361) projected
  line L621 (-93.8375, 298.45) -> (-59.186, 298.45) projected
  line L622 (-59.186, 298.45) -> (-76.5118, 281.1243) projected
  line L623 (-76.5118, 281.1243) -> (-93.8375, 298.45) projected
  line L624 (-127.5196, 273.9401) -> (-105.6078, 252.0282) projected
  line L625 (-105.6078, 252.0282) -> (-127.5196, 230.1164) projected
  line L626 (-127.5196, 230.1164) -> (-146.05, 248.6468) projected
  line L627 (-146.05, 248.6468) -> (-146.05, 255.4097) projected
  line L628 (-146.05, 255.4097) -> (-127.5196, 273.9401) projected
  line L629 (-76.5118, 222.9322) -> (-54.6, 201.0204) projected
  line L630 (-54.6, 201.0204) -> (-76.5118, 179.1086) projected
  line L631 (-76.5118, 179.1086) -> (-98.4236, 201.0204) projected
  line L632 (-98.4236, 201.0204) -> (-76.5118, 222.9322) projected
  line L633 (-127.5196, 128.1007) -> (-149.4315, 150.0125) projected
  line L634 (-149.4315, 150.0125) -> (-127.5196, 171.9243) projected
  line L635 (-127.5196, 171.9243) -> (-105.6078, 150.0125) projected
  line L636 (-105.6078, 150.0125) -> (-127.5196, 128.1007) projected
  line L637 (-51.0079, 197.4283) -> (-29.096, 175.5165) projected
  line L638 (-29.096, 175.5165) -> (-51.0079, 153.6046) projected
  line L639 (-51.0079, 153.6046) -> (-72.9197, 175.5165) projected
  line L640 (-72.9197, 175.5165) -> (-51.0079, 197.4283) projected
  line L641 (-127.5196, 120.9165) -> (-105.6078, 99.0047) projected
  line L642 (-105.6078, 99.0047) -> (-127.5196, 77.0928) projected
  line L643 (-127.5196, 77.0928) -> (-149.4315, 99.0047) projected
  line L644 (-149.4315, 99.0047) -> (-127.5196, 120.9165) projected
  line L645 (-178.5275, 120.9165) -> (-156.6157, 99.0047) projected
  line L646 (-156.6157, 99.0047) -> (-178.5275, 77.0928) projected
  line L647 (-178.5275, 77.0928) -> (-200.4393, 99.0047) projected
  line L648 (-200.4393, 99.0047) -> (-178.5275, 120.9165) projected
  line L649 (-102.0157, 0.5811) -> (-123.9275, 22.4929) projected
  line L650 (-123.9275, 22.4929) -> (-102.0157, 44.4047) projected
  line L651 (-102.0157, 44.4047) -> (-80.1039, 22.4929) projected
  line L652 (-80.1039, 22.4929) -> (-102.0157, 0.5811) projected
  line L653 (-25.5039, 26.085) -> (-47.4158, 47.9968) projected
  line L654 (-47.4158, 47.9968) -> (-25.5039, 69.9086) projected
  line L655 (-25.5039, 69.9086) -> (-3.5921, 47.9968) projected
  line L656 (-3.5921, 47.9968) -> (-25.5039, 26.085) projected
  line L657 (25.5039, -24.9229) -> (3.5921, -3.011) projected
  line L658 (3.5921, -3.011) -> (25.5039, 18.9008) projected
  line L659 (25.5039, 18.9008) -> (47.4158, -3.011) projected
  line L660 (47.4158, -3.011) -> (25.5039, -24.9229) projected
  line L661 (-51.0079, -57.611) -> (-29.096, -79.5228) projected
  line L662 (-29.096, -79.5228) -> (-51.0079, -101.4346) projected
  line L663 (-51.0079, -101.4346) -> (-72.9197, -79.5228) projected
  line L664 (-72.9197, -79.5228) -> (-51.0079, -57.611) projected
  line L665 (-76.5118, -32.1071) -> (-54.6, -54.0189) projected
  line L666 (-54.6, -54.0189) -> (-76.5118, -75.9307) projected
  line L667 (-76.5118, -75.9307) -> (-98.4236, -54.0189) projected
  line L668 (-98.4236, -54.0189) -> (-76.5118, -32.1071) projected
  line L669 (-131.1117, -28.515) -> (-153.0236, -50.4268) projected
  line L670 (-153.0236, -50.4268) -> (-174.9354, -28.515) projected
  line L671 (-174.9354, -28.515) -> (-153.0236, -6.6031) projected
  line L672 (-153.0236, -6.6031) -> (-131.1117, -28.515) projected
  line L673 (-127.5196, -83.1149) -> (-105.6078, -105.0267) projected
  line L674 (-105.6078, -105.0267) -> (-127.5196, -126.9386) projected
  line L675 (-127.5196, -126.9386) -> (-149.4315, -105.0267) projected
  line L676 (-149.4315, -105.0267) -> (-127.5196, -83.1149) projected
  line L677 (0, 153.6046) -> (-21.9118, 175.5165) projected
  line L678 (-21.9118, 175.5165) -> (0, 197.4283) projected
  line L679 (0, 197.4283) -> (21.9118, 175.5165) projected
  line L680 (21.9118, 175.5165) -> (0, 153.6046) projected
  line L681 (-284.1353, 124.5086) -> (-298.45, 110.1939) projected
  line L682 (-298.45, 110.1939) -> (-298.45, 138.8233) projected
  line L683 (-298.45, 138.8233) -> (-284.1353, 124.5086) projected
  line L684 (-204.0314, 95.4126) -> (-182.1196, 73.5007) projected
  line L685 (-182.1196, 73.5007) -> (-204.0246, 51.5957) projected
  line L686 (-204.0246, 51.5957) -> (-225.9331, 73.5109) projected
  line L687 (-225.9331, 73.5109) -> (-204.0314, 95.4126) projected
  line L688 (-255.0393, 44.4047) -> (-233.1274, 22.4929) projected
  line L689 (-233.1274, 22.4929) -> (-255.0393, 0.5811) projected
  line L690 (-255.0393, 0.5811) -> (-276.9511, 22.4929) projected
  line L691 (-276.9511, 22.4929) -> (-255.0393, 44.4047) projected
  line L692 (-280.5432, 18.9008) -> (-258.6314, -3.011) projected
  line L693 (-258.6314, -3.011) -> (-280.5432, -24.9229) projected
  line L694 (-280.5432, -24.9229) -> (-298.45, -7.0161) projected
  line L695 (-298.45, -7.0161) -> (-298.45, 0.994) projected
  line L696 (-298.45, 0.994) -> (-280.5432, 18.9008) projected
  line L697 (-200.4393, -3.011) -> (-178.5275, 18.9008) projected
  line L698 (-178.5275, 18.9008) -> (-156.6157, -3.011) projected
  line L699 (-156.6157, -3.011) -> (-178.5275, -24.9229) projected
  line L700 (-178.5275, -24.9229) -> (-200.4393, -3.011) projected
  line L701 (-284.1353, -79.5228) -> (-298.45, -93.8375) projected
  line L702 (-298.45, -93.8375) -> (-298.45, -65.2081) projected
  line L703 (-298.45, -65.2081) -> (-284.1353, -79.5228) projected
  line L704 (-284.1353, -28.515) -> (-298.45, -42.8297) projected
  line L705 (-298.45, -42.8297) -> (-298.45, -14.2003) projected
  line L706 (-298.45, -14.2003) -> (-284.1353, -28.515) projected
  line L707 (-255.0393, -6.6031) -> (-233.1274, -28.515) projected
  line L708 (-233.1274, -28.515) -> (-255.0393, -50.4268) projected
  line L709 (-255.0393, -50.4268) -> (-276.9511, -28.515) projected
  line L710 (-276.9511, -28.515) -> (-255.0393, -6.6031) projected
  line L711 (-280.5432, 69.9086) -> (-258.6314, 47.9968) projected
  line L712 (-258.6314, 47.9968) -> (-280.5432, 26.085) projected
  line L713 (-280.5432, 26.085) -> (-298.45, 43.9918) projected
  line L714 (-298.45, 43.9918) -> (-298.45, 52.0018) projected
  line L715 (-298.45, 52.0018) -> (-280.5432, 69.9086) projected
  line L716 (-178.5275, 69.9086) -> (-156.6157, 47.9968) projected
  line L717 (-156.6157, 47.9968) -> (-178.5246, 26.0879) projected
  line L718 (-178.5246, 26.0879) -> (-200.4331, 48.0031) projected
  line L719 (-200.4331, 48.0031) -> (-178.5275, 69.9086) projected
  line L720 (-280.5432, 120.9165) -> (-258.6314, 99.0047) projected
  line L721 (-258.6314, 99.0047) -> (-280.5432, 77.0928) projected
  line L722 (-280.5432, 77.0928) -> (-298.45, 94.9996) projected
  line L723 (-298.45, 94.9996) -> (-298.45, 103.0097) projected
  line L724 (-298.45, 103.0097) -> (-280.5432, 120.9165) projected
  arc A16 (-222.25, 146.05) -> (-210.7066, 146.9294) centre (-222.25, 222.25) ccw projected
  line L725 (-210.7066, 146.9294) -> (-229.5353, 128.1007) projected
  line L726 (-229.5353, 128.1007) -> (-247.4846, 146.05) projected
  line L727 (-247.4846, 146.05) -> (-222.25, 146.05) projected
  line L728 (-153.0236, -57.611) -> (-131.1117, -79.5228) projected
  line L729 (-131.1117, -79.5228) -> (-153.0236, -101.4346) projected
  line L730 (-153.0236, -101.4346) -> (-174.9354, -79.5228) projected
  line L731 (-174.9354, -79.5228) -> (-153.0236, -57.611) projected
  line L732 (-127.5196, -75.9307) -> (-149.4315, -54.0189) projected
  line L733 (-149.4315, -54.0189) -> (-127.5196, -32.1071) projected
  line L734 (-127.5196, -32.1071) -> (-105.6078, -54.0189) projected
  line L735 (-105.6078, -54.0189) -> (-127.5196, -75.9307) projected
  line L736 (-102.0157, -6.6031) -> (-80.1039, -28.515) projected
  line L737 (-80.1039, -28.515) -> (-102.0157, -50.4268) projected
  line L738 (-102.0157, -50.4268) -> (-123.9275, -28.515) projected
  line L739 (-123.9275, -28.515) -> (-102.0157, -6.6031) projected
  line L740 (-51.0079, -50.4268) -> (-72.9197, -28.515) projected
  line L741 (-72.9197, -28.515) -> (-51.0079, -6.6031) projected
  line L742 (-51.0079, -6.6031) -> (-29.096, -28.515) projected
  line L743 (-29.096, -28.515) -> (-51.0079, -50.4268) projected
  line L744 (-25.5039, -24.9229) -> (-47.4158, -3.011) projected
  line L745 (-47.4158, -3.011) -> (-25.5039, 18.9008) projected
  line L746 (-25.5039, 18.9008) -> (-3.5921, -3.011) projected
  line L747 (-3.5921, -3.011) -> (-25.5039, -24.9229) projected
  line L748 (0, 95.4126) -> (21.9118, 73.5007) projected
  line L749 (21.9118, 73.5007) -> (0, 51.5889) projected
  line L750 (0, 51.5889) -> (-21.9118, 73.5007) projected
  line L751 (-21.9118, 73.5007) -> (0, 95.4126) projected
  line L752 (-54.6, 47.9968) -> (-76.5118, 26.085) projected
  line L753 (-76.5118, 26.085) -> (-98.4236, 47.9968) projected
  line L754 (-98.4236, 47.9968) -> (-76.5118, 69.9086) projected
  line L755 (-76.5118, 69.9086) -> (-54.6, 47.9968) projected
  line L756 (-153.0236, 95.4126) -> (-131.1117, 73.5007) projected
  line L757 (-131.1117, 73.5007) -> (-153.0236, 51.5889) projected
  line L758 (-153.0236, 51.5889) -> (-174.9354, 73.5007) projected
  line L759 (-174.9354, 73.5007) -> (-153.0236, 95.4126) projected
  line L760 (-153.0236, 146.4204) -> (-131.1117, 124.5086) projected
  line L761 (-131.1117, 124.5086) -> (-153.0236, 102.5968) projected
  line L762 (-153.0236, 102.5968) -> (-174.9354, 124.5086) projected
  line L763 (-174.9354, 124.5086) -> (-153.0236, 146.4204) projected
  line L764 (-25.5039, 171.9243) -> (-3.5921, 150.0125) projected
  line L765 (-3.5921, 150.0125) -> (-25.5039, 128.1007) projected
  line L766 (-25.5039, 128.1007) -> (-47.4158, 150.0125) projected
  line L767 (-47.4158, 150.0125) -> (-25.5039, 171.9243) projected
  line L768 (-102.0157, 197.4283) -> (-80.1039, 175.5165) projected
  line L769 (-80.1039, 175.5165) -> (-102.0157, 153.6046) projected
  line L770 (-102.0157, 153.6046) -> (-123.9275, 175.5165) projected
  line L771 (-123.9275, 175.5165) -> (-102.0157, 197.4283) projected
  line L772 (-127.5196, 222.9322) -> (-105.6078, 201.0204) projected
  line L773 (-105.6078, 201.0204) -> (-127.5196, 179.1086) projected
  line L774 (-127.5196, 179.1086) -> (-149.1495, 200.7384) projected
  arc A17 (-149.1495, 200.7384) -> (-148.9209, 201.531) centre (-222.25, 222.25) ccw projected
  line L775 (-148.9209, 201.531) -> (-127.5196, 222.9322) projected
  line L776 (-102.0157, 248.4361) -> (-80.1039, 226.5243) projected
  line L777 (-80.1039, 226.5243) -> (-102.0157, 204.6125) projected
  line L778 (-102.0157, 204.6125) -> (-123.9275, 226.5243) projected
  line L779 (-123.9275, 226.5243) -> (-102.0157, 248.4361) projected
  line L780 (-123.9275, 277.5322) -> (-103.0097, 298.45) projected
  line L781 (-103.0097, 298.45) -> (-101.0217, 298.45) projected
  line L782 (-101.0217, 298.45) -> (-80.1039, 277.5322) projected
  line L783 (-80.1039, 277.5322) -> (-102.0157, 255.6203) projected
  line L784 (-102.0157, 255.6203) -> (-123.9275, 277.5322) projected
  line L785 (-25.5039, 273.9401) -> (-3.5921, 252.0282) projected
  line L786 (-3.5921, 252.0282) -> (-25.5039, 230.1164) projected
  line L787 (-25.5039, 230.1164) -> (-47.4158, 252.0282) projected
  line L788 (-47.4158, 252.0282) -> (-25.5039, 273.9401) projected
  line L789 (25.5039, 230.1164) -> (3.5921, 252.0282) projected
  line L790 (3.5921, 252.0282) -> (25.5039, 273.9401) projected
  line L791 (25.5039, 273.9401) -> (47.4158, 252.0282) projected
  line L792 (47.4158, 252.0282) -> (25.5039, 230.1164) projected
  line L793 (76.5118, 273.9401) -> (98.4236, 252.0282) projected
  line L794 (98.4236, 252.0282) -> (76.5118, 230.1164) projected
  line L795 (76.5118, 230.1164) -> (54.6, 252.0282) projected
  line L796 (54.6, 252.0282) -> (76.5118, 273.9401) projected
  line L797 (25.5039, -134.1228) -> (47.4158, -156.0346) projected
  line L798 (47.4158, -156.0346) -> (25.5039, -177.9464) projected
  line L799 (25.5039, -177.9464) -> (3.5921, -156.0346) projected
  line L800 (3.5921, -156.0346) -> (25.5039, -134.1228) projected
  line L801 (102.0157, -152.4425) -> (80.1039, -130.5307) projected
  line L802 (80.1039, -130.5307) -> (102.0157, -108.6189) projected
  line L803 (102.0157, -108.6189) -> (123.9275, -130.5307) projected
  line L804 (123.9275, -130.5307) -> (102.0157, -152.4425) projected
  line L805 (146.05, 241.4626) -> (146.05, 222.25) projected
  arc A18 (146.05, 222.25) -> (146.9294, 210.7066) centre (222.25, 222.25) ccw projected
  line L806 (146.9294, 210.7066) -> (131.1117, 226.5243) projected
  line L807 (131.1117, 226.5243) -> (146.05, 241.4626) projected
  line L808 (-21.9118, 124.5086) -> (0, 146.4204) projected
  line L809 (0, 146.4204) -> (21.9118, 124.5086) projected
  line L810 (21.9118, 124.5086) -> (0, 102.5968) projected
  line L811 (0, 102.5968) -> (-21.9118, 124.5086) projected
  line L812 (102.0157, 153.6046) -> (80.1039, 175.5165) projected
  line L813 (80.1039, 175.5165) -> (102.0157, 197.4283) projected
  line L814 (102.0157, 197.4283) -> (123.9275, 175.5165) projected
  line L815 (123.9275, 175.5165) -> (102.0157, 153.6046) projected
  line L816 (51.0079, 44.4047) -> (72.9197, 22.4929) projected
  line L817 (72.9197, 22.4929) -> (51.0079, 0.5811) projected
  line L818 (51.0079, 0.5811) -> (29.096, 22.4929) projected
  line L819 (29.096, 22.4929) -> (51.0079, 44.4047) projected
  line L820 (76.5118, 120.9165) -> (98.4236, 99.0047) projected
  line L821 (98.4236, 99.0047) -> (76.5118, 77.0928) projected
  line L822 (76.5118, 77.0928) -> (54.6, 99.0047) projected
  line L823 (54.6, 99.0047) -> (76.5118, 120.9165) projected
  line L824 (178.5275, 77.0928) -> (156.6157, 99.0047) projected
  line L825 (156.6157, 99.0047) -> (178.5275, 120.9165) projected
  line L826 (178.5275, 120.9165) -> (200.4393, 99.0047) projected
  line L827 (200.4393, 99.0047) -> (178.5275, 77.0928) projected
  line L828 (127.5196, 69.9086) -> (149.4315, 47.9968) projected
  line L829 (149.4315, 47.9968) -> (127.5196, 26.085) projected
  line L830 (127.5196, 26.085) -> (105.6078, 47.9968) projected
  line L831 (105.6078, 47.9968) -> (127.5196, 69.9086) projected
  line L832 (102.0157, -101.4346) -> (80.1039, -79.5228) projected
  line L833 (80.1039, -79.5228) -> (102.0157, -57.611) projected
  line L834 (102.0157, -57.611) -> (123.9275, -79.5228) projected
  line L835 (123.9275, -79.5228) -> (102.0157, -101.4346) projected
  line L836 (174.933, 22.4952) -> (159.5933, 7.1508) projected
  line L837 (159.5933, 7.1508) -> (153.0236, 0.5811) projected
  line L838 (153.0236, 0.5811) -> (131.1117, 22.4929) projected
  line L839 (131.1117, 22.4929) -> (153.0236, 44.4047) projected
  line L840 (153.0236, 44.4047) -> (174.933, 22.4952) projected
  line L841 (153.0236, -6.6031) -> (174.9354, -28.515) projected
  line L842 (174.9354, -28.515) -> (153.0236, -50.4268) projected
  line L843 (153.0236, -50.4268) -> (131.1117, -28.515) projected
  line L844 (131.1117, -28.515) -> (153.0236, -6.6031) projected
  line L845 (229.5353, -24.9229) -> (207.6235, -3.011) projected
  line L846 (207.6235, -3.011) -> (229.5353, 18.9008) projected
  line L847 (229.5353, 18.9008) -> (251.4472, -3.011) projected
  line L848 (251.4472, -3.011) -> (229.5353, -24.9229) projected
  line L849 (255.0393, 0.5811) -> (233.1274, 22.4929) projected
  line L850 (233.1274, 22.4929) -> (255.0393, 44.4047) projected
  line L851 (255.0393, 44.4047) -> (276.9511, 22.4929) projected
  line L852 (276.9511, 22.4929) -> (255.0393, 0.5811) projected
  line L853 (280.5432, 77.0928) -> (258.6314, 99.0047) projected
  line L854 (258.6314, 99.0047) -> (280.5432, 120.9165) projected
  line L855 (280.5432, 120.9165) -> (298.45, 103.0097) projected
  line L856 (298.45, 103.0097) -> (298.45, 94.9996) projected
  line L857 (298.45, 94.9996) -> (280.5432, 77.0928) projected
  line L858 (284.1353, 124.5086) -> (298.45, 138.8233) projected
  line L859 (298.45, 138.8233) -> (298.45, 110.1939) projected
  line L860 (298.45, 110.1939) -> (284.1353, 124.5086) projected
  line L861 (21.9118, -283.5542) -> (7.0161, -298.45) projected
  line L862 (7.0161, -298.45) -> (-7.0161, -298.45) projected
  line L863 (-7.0161, -298.45) -> (-21.9118, -283.5542) projected
  line L864 (-21.9118, -283.5542) -> (0, -261.6424) projected